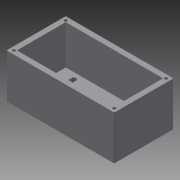
# Autodesk Inventor part: Solenoids_holder
Saved by Autodesk Inventor 2015 (Build 190159000, 159)
## iProperties
Created: 2015-11-10
Part Number: Solenoids_holder
Material: Generic
Document SubType Name: Modeling
Designer: Lauszus
Density: 1 g/cm^3
Appearance: Default
Author: Lauszus
Autodesk Inventor part; units mm, degrees
ref_plane "YZ Plane" through (0, 0, 0) normal (1, 0, 0) x (0, 1, 0)
ref_plane "XZ Plane" through (0, 0, 0) normal (0, 1, 0) x (-1, 0, 0)
ref_plane "XY Plane" through (0, 0, 0) normal (0, 0, 1) x (1, 0, 0)
sketch "Sketch1" plane through (0, 0, 0) normal (0, 0, 1) x (1, 0, 0)
  line L0 (-42.0539, 29.2948) -> (30.7461, 29.2948)
  line L1 (30.7461, 29.2948) -> (30.7461, -10.7052)
  line L2 (30.7461, -10.7052) -> (-42.0539, -10.7052)
  line L3 (-42.0539, -10.7052) -> (-42.0539, 29.2948)
  point P0 (0, 0)
  dimension "d0" = 72.8
  dimension "d1" = 40
  constraints: 8 end point, 2 parallel, 1 horizontal, 1 perpendicular
  measures "d0" distance of L0.start L0.end
  measures "d1" distance of L2.end L0.start
extrude "Extrusion1" add sketch "Sketch1" along normal blind 30
shell "Shell2" thickness 3.5 removed faces 1 at (-17.7872, 15.9615, 30)
sketch "Sketch4" plane through (0, 0, 30) normal (0, 0, 1) x (1, 0, 0)
  circle A0 centre (-39.5539, 26.7948) radius 1
  line L0 (30.7461, 29.2948) -> (-42.0539, 29.2948) projected
  line L1 (-42.0539, 29.2948) -> (-42.0539, -10.7052) projected
  line L2 (-5.6539, 34.5623) -> (-5.6539, 23.6795)
  circle A1 centre (28.2461, 26.7948) radius 1
  line L3 (36.847, 9.2948) -> (23.7014, 9.2948)
  circle A2 centre (28.2461, -8.2052) radius 1
  circle A3 centre (-39.5539, -8.2052) radius 1
  point P0 (0, 0)
  dimension "d26" = 2
  dimension "d27" = 2.5
  dimension "d28" = 2.5
  constraints: 4 centre point, 4 end point, 3 symmetric about line, 1 horizontal, 1 vertical, 3 other
  measures "d26" diameter of A0
  measures "d27" distance from line of A0.centre L0
  measures "d28" distance from line of A0.centre L1
extrude "Extrusion4" cut sketch "Sketch4" against normal blind 4
fillet "Fillet1" radius 0.4 8 edges at (-42.0539, 29.2948, 15) (-42.0539, -10.7052, 15) (30.7461, -10.7052, 15) (30.7461, 29.2948, 15) (-5.6539, -10.7052, 0) (30.7461, 9.2948, 0) (-5.6539, 29.2948, 0) (-42.0539, 9.2948, 0)
sketch "Sketch5" plane through (0, 0, 0) normal (0, 0, -1) x (-1, 0, 0)
  line L0 (41.6539, -10.7052) -> (-30.3461, -10.7052) projected
  line L1 (5.6539, -10.7052) -> (5.6539, 29.2948)
  line L2 (-30.3461, 29.2948) -> (41.6539, 29.2948) projected
  circle A0 centre (22.8539, 9.2948) radius 9.5
  circle A1 centre (-11.5461, 10.9904) radius 9.5
  line L3 (-17.5461, 8.6249) -> (-17.5461, -1.3751) construction
  line L4 (-19.0461, 8.6249) -> (-19.0461, -1.3751)
  line L5 (-16.0461, -1.3751) -> (-16.0461, 8.6249)
  arc A2 (-16.0461, 8.6249) -> (-19.0461, 8.6249) centre (-17.5461, 8.6249) ccw
  arc A3 (-19.0461, -1.3751) -> (-16.0461, -1.3751) centre (-17.5461, -1.3751) ccw
  line L6 (-5.5461, 13.3558) -> (-5.5461, 23.3558) construction
  line L7 (-4.0461, 13.3558) -> (-4.0461, 23.3558)
  line L8 (-7.0461, 23.3558) -> (-7.0461, 13.3558)
  arc A4 (-7.0461, 13.3558) -> (-4.0461, 13.3558) centre (-5.5461, 13.3558) ccw
  arc A5 (-4.0461, 23.3558) -> (-7.0461, 23.3558) centre (-5.5461, 23.3558) ccw
  line L9 (16.8539, 6.9294) -> (16.8539, -3.0706) construction
  line L10 (15.3539, 6.9294) -> (15.3539, -3.0706)
  line L11 (18.3539, -3.0706) -> (18.3539, 6.9294)
  arc A6 (18.3539, 6.9294) -> (15.3539, 6.9294) centre (16.8539, 6.9294) ccw
  arc A7 (15.3539, -3.0706) -> (18.3539, -3.0706) centre (16.8539, -3.0706) ccw
  line L12 (28.8539, 11.6603) -> (28.8539, 21.6603) construction
  line L13 (30.3539, 11.6603) -> (30.3539, 21.6603)
  line L14 (27.3539, 21.6603) -> (27.3539, 11.6603)
  arc A8 (27.3539, 11.6603) -> (30.3539, 11.6603) centre (28.8539, 11.6603) ccw
  arc A9 (30.3539, 21.6603) -> (27.3539, 21.6603) centre (28.8539, 21.6603) ccw
  point P0 (0, 0)
  point P1 (-17.5461, 3.6249)
  point P2 (-5.5461, 18.3558)
  point P3 (16.8539, 1.9294)
  point P4 (28.8539, 16.6603)
  dimension "d32" = 19
  dimension "d33" = 19
  dimension "d34" = 5
  dimension "d35" = 3
  dimension "d36" = 5
  dimension "d37" = 3
  dimension "d38" = 5
  dimension "d39" = 3
  dimension "d40" = 5
  dimension "d41" = 3
  dimension "d42" = 17.2
  dimension "d43" = 17.2
  dimension "d44" = 6
  dimension "d45" = 12
  dimension "d46" = 6
  dimension "d47" = 12
  constraints: 34 end point, 20 point on circle, 16 tangent, 10 centre point, 7 parallel, 6 midpoint, 1 vertical
  measures "d32" diameter of A0
  measures "d33" diameter of A1
  measures "d34" distance of A1.start L3.end
  measures "d35" diameter of A3
  measures "d36" distance of A1.end L6.end
  measures "d37" diameter of A5
  measures "d38" distance of A0.start L9.end
  measures "d39" diameter of A7
  measures "d40" distance of A0.end L12.end
  measures "d41" diameter of A9
  measures "d42" distance from line of L1 A0.centre
  measures "d43" distance from line of A1.centre L1
  measures "d44" horizontal distance of A0.centre A0.start
  measures "d45" horizontal distance of A0.start A0.end
  measures "d46" horizontal distance of A1.centre A1.end
  measures "d47" horizontal distance of A1.end A1.start
extrude "Extrusion5" cut sketch "Sketch5" against normal through all contours L13 A8 L14 A0 | A0 L14 A9 L13 | L11 A7 L10 A0 | A0 L10 A6 L11 | L7 A4 L8 A1 | A1 L8 A5 L7 | L5 A3 L4 A1 | A1 L4 A2 L5
body "Solid1"
